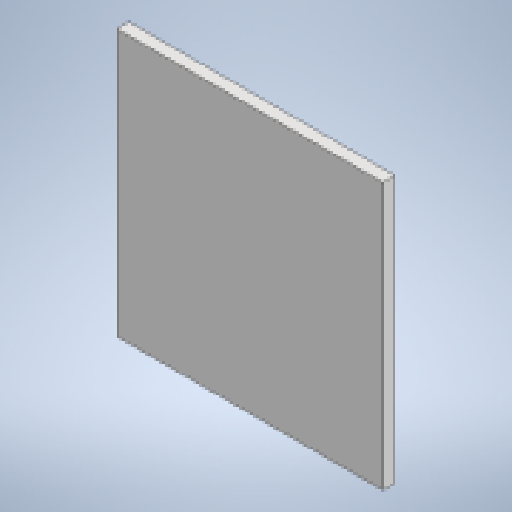
# Autodesk Inventor part: Parte deslizante
Saved by Autodesk Inventor 2024 (Build 280153000, 153)
## iProperties
Created: 2025-03-02
Part Number: Parte deslizante
Material: Genérico
Document SubType Name: Modeling
Designer: sergi
Density: 1 g/cm^3
Appearance: Valor por defecto
Author: sergi
Autodesk Inventor part; units mm, degrees
ref_plane "YZ Plane" through (0, 0, 0) normal (1, 0, 0) x (0, 1, 0)
ref_plane "XZ Plane" through (0, 0, 0) normal (0, 1, 0) x (-1, 0, 0)
ref_plane "XY Plane" through (0, 0, 0) normal (0, 0, 1) x (1, 0, 0)
sketch "Boceto1" plane through (0, 0, 0) normal (0, 0, 1) x (1, 0, 0)
  line L0 (-32, -32) -> (32, -32)
  line L1 (32, -32) -> (32, 32)
  line L2 (32, 32) -> (-32, 32)
  line L3 (-32, 32) -> (-32, -32)
  line L4 (-32, -32) -> (32, 32) construction
  line L5 (32, -32) -> (-32, 32) construction
  point P0 (0, 0)
  dimension "d0" = 64
  dimension "d1" = 64
  constraints: 12 end point, 2 midpoint, 2 parallel, 1 horizontal, 1 perpendicular
  measures "d0" distance of L2.end L1.end
  measures "d1" distance of L1.end L0.end
extrude "Extrusión1" add sketch "Boceto1" along normal blind 3
sketch "Boceto2" plane through (32, -32, 0) normal (1, 0, 0) x (0, 0, -1)
  line L0 (-74, 16.5) -> (1, 16.5) projected
  arc A0 (1, 10.5) -> (1, 16.5) centre (1, 13.5) ccw projected
  line L1 (1, 10.5) -> (-74, 10.5) projected
  line L2 (-74, -4.5) -> (-74, 10.5) projected
  line L3 (7, -4.5) -> (-74, -4.5) projected
  line L4 (7, -4.5) -> (7, 68.5) projected
  line L5 (7, 68.5) -> (-74, 68.5) projected
  line L6 (-74, 53.5) -> (-74, 68.5) projected
  line L7 (-74, 53.5) -> (1, 53.5) projected
  arc A1 (1, 47.5) -> (1, 53.5) centre (1, 50.5) ccw projected
  line L8 (1, 47.5) -> (-74, 47.5) projected
  line L9 (-74, 16.5) -> (-74, 47.5) projected
  line L10 (0, 0) -> (0, 64) projected
  line L11 (0, 64) -> (-3, 64) projected
  line L12 (-3, 0) -> (-3, 64) projected
  line L13 (0, 0) -> (-3, 0) projected
  line L14 (0, 47.5) -> (-3, 47.5)
  line L15 (-3, 47.5) -> (-3, 53.5)
  line L16 (-3, 53.5) -> (0, 53.5)
  line L17 (0, 53.5) -> (0, 47.5)
  line L18 (0, 47.7) -> (-3, 47.7)
  line L19 (-2.8, 47.7) -> (-2.8, 53.3)
  line L20 (-3, 53.3) -> (0, 53.3)
  line L21 (-0.2, 53.3) -> (-0.2, 47.7)
  point P0 (0, 32)
  dimension "d4" = 0.2
  constraints: 16 end point, 12 point on line, 4 parallel, 2 perpendicular, 1 horizontal
  measures "d4" distance between parallel lines of L17 L21
extrude "Extrusión2" add sketch "Boceto2" along normal blind 10 contours L12 L20 L19 L18 | L18 L21 L20 L10 | L19 L20 L21 L18
sketch "Boceto3" plane through (42, -32, 0) normal (1, 0, 0) x (0, 0, -1)
  line L0 (-3, 53.3) -> (-3, 47.7) projected
  line L1 (-3, 47.7) -> (0, 47.7) projected
  line L2 (0, 47.7) -> (0, 53.3) projected
  line L3 (0, 53.3) -> (-3, 53.3) projected
  line L4 (0, 47.7) -> (-3, 53.3)
  circle A0 centre (-1.5, 50.5) radius 5
  line L5 (-3, 53.3) -> (-3, 55.2697)
  line L6 (-3, 47.7) -> (0, 47.7)
  line L7 (0, 47.7) -> (0, 53.3)
  line L8 (0, 53.3) -> (-3, 53.3)
  line L9 (-3, 53.3) -> (-3, 47.7)
  line L10 (-3, 47.7) -> (-3, 42)
  point P0 (0, 32)
  point P1 (-3, 45.7303)
  dimension "d7" = 10
  constraints: 14 end point, 2 parallel, 1 horizontal, 1 midpoint, 1 perpendicular, 1 vertical, 3 other
extrude "Extrusión3" add sketch "Boceto3" along normal blind 3 contours L4 L1 L0 | L5 A0 L10 L1 L2 L3 | L3 L2 L4
ref_plane "Plano de trabajo1" through (0, -32, 3) normal (1, 0, 0) x (0, 0, -1)
ref_plane "Plano de trabajo2" through (-32, 0, 0) normal (0, 1, 0) x (1, 0, 0)
mirror "Simetría1" about plane through (-32, 0, 0) normal (0, 1, 0) of "Extrusión2", "Extrusión3"
mirror "Simetría2" about plane through (0, -32, 3) normal (1, 0, 0) of "Extrusión2", "Simetría1", "Extrusión3"
